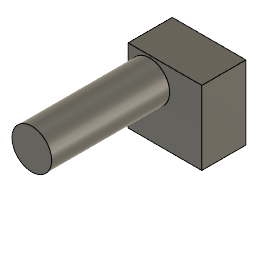
heltec-wp-knopf (Autodesk Fusion 360 design; units mm, degrees)
Autodesk Fusion 360 part; units mm, degrees
sketch "Skizze1" plane through (0, 0, 0) normal (0, 1, 0) x (1, 0, 0)
  line L0 (-7.3758, -5.9007) -> (-2.3758, -5.9007)
  line L1 (-2.3758, -5.9007) -> (-2.3758, -0.9007)
  line L2 (-2.3758, -0.9007) -> (-7.3758, -0.9007)
  line L3 (-7.3758, -0.9007) -> (-7.3758, -5.9007)
  circle A0 centre (-5.9, -4.4) radius 1.35
  dimension "d1" = 5
  dimension "d2" = 5
  dimension "d8" = 2.7
  constraint horizontal L0
  constraint vertical L1
  constraint horizontal L2
  constraint vertical L3
  measures "d1" distance of L0.start L0.end
  measures "d2" distance of L0.start L2.end
  measures "d8" diameter of A0
extrude "Extrusion1" add sketch "Skizze1" along normal blind 3 contours L0 L1 L2 L3 | A0
sketch "Skizze3" plane through (0, 0, 0) normal (0, -1, 0) x (1, 0, 0)
  line L0 (-7.3758, 5.9007) -> (-7.3758, 0.9007)
  line L1 (-7.3758, 0.9007) -> (-2.3758, 0.9007)
  line L2 (-2.3758, 0.9007) -> (-2.3758, 5.9007)
  line L3 (-2.3758, 5.9007) -> (-7.3758, 5.9007)
  circle A0 centre (-5.9, 4.4) radius 1.35
  dimension "d9" = 2.7
  measures "d9" diameter of A0
extrude "Extrusion3" add sketch "Skizze3" along normal blind 8 contours A0
